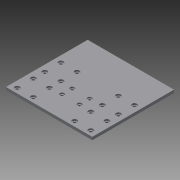
# Autodesk Inventor part: mic6_plate
Saved by Autodesk Inventor 2014 (Build 180170000, 170)
## iProperties
Created: 2014-08-09
Part Number: mic6_plate
Material: Generic
Document SubType Name: Modeling
Designer: Matthew
Density: 1 g/cm^3
Appearance: Default
Mass: 265.145 g
Surface Area: 932.163 cm^2
Volume: 265.145 cm^3
Author: Matthew
Autodesk Inventor part; units mm, degrees
ref_plane "YZ Plane" through (0, 0, 0) normal (1, 0, 0) x (0, 1, 0)
ref_plane "XZ Plane" through (0, 0, 0) normal (0, 1, 0) x (-1, 0, 0)
ref_plane "XY Plane" through (0, 0, 0) normal (0, 0, 1) x (1, 0, 0)
sketch "Sketch1" plane through (0, 0, 0) normal (0, 1, 0) x (-1, 0, 0)
  line L0 (93.9, 88.9) -> (-93.9, 88.9)
  line L1 (-93.9, 88.9) -> (-93.9, -88.9)
  line L2 (-93.9, -88.9) -> (93.9, -88.9)
  line L3 (93.9, -88.9) -> (93.9, 88.9)
  line L4 (93.9, 88.9) -> (-93.9, -88.9) construction
  line L5 (-93.9, 88.9) -> (93.9, -88.9) construction
  point P0 (0, 0)
  dimension "d0" = 187.8
  dimension "d1" = 177.8
  constraints: 12 end point, 2 midpoint, 2 parallel, 1 horizontal, 1 perpendicular
  measures "d0" distance of L2.end L1.end
  measures "d1" distance of L0.end L1.end
extrude "Extrusion1" add sketch "Sketch1" along normal blind 6.35
sketch "Sketch3" plane through (0, 6.35, 0) normal (0, 1, 0) x (1, 0, 0)
  line L0 (-93.9, 88.9) -> (-93.9, -88.9)
  line L1 (93.9, 88.9) -> (-93.9, 88.9)
  line L2 (-86.5034, 24.275) -> (-86.5034, -25.725) construction
  line L3 (-86.5034, -25.725) -> (-38.5034, -25.725) construction
  line L4 (-38.5034, -25.725) -> (-38.5034, 24.275) construction
  line L5 (-38.5034, 24.275) -> (-86.5034, 24.275) construction
  line L6 (38.5034, 24.275) -> (38.5034, -25.725) construction
  line L7 (38.5034, -25.725) -> (86.5034, -25.725) construction
  line L8 (86.5034, -25.725) -> (86.5034, 24.275) construction
  line L9 (86.5034, 24.275) -> (38.5034, 24.275) construction
  line L10 (-86.5034, -35.725) -> (-86.5034, -85.725) construction
  line L11 (-86.5034, -85.725) -> (-38.5034, -85.725) construction
  line L12 (-38.5034, -85.725) -> (-38.5034, -35.725) construction
  line L13 (-38.5034, -35.725) -> (-86.5034, -35.725) construction
  line L14 (38.5034, -35.725) -> (38.5034, -85.725) construction
  line L15 (38.5034, -85.725) -> (86.5034, -85.725) construction
  line L16 (86.5034, -85.725) -> (86.5034, -35.725) construction
  line L17 (86.5034, -35.725) -> (38.5034, -35.725) construction
  line L18 (-24, -13.225) -> (24, -13.225) construction
  line L19 (24, -13.225) -> (24, -48.225) construction
  line L20 (24, -48.225) -> (-24, -48.225) construction
  line L21 (-24, -48.225) -> (-24, -13.225) construction
  line L22 (93.9, -88.9) -> (93.9, 88.9) projected
  line L23 (-93.9, -88.9) -> (93.9, -88.9) projected
  point P0 (-133.35, 152.4)
  point P1 (-152.4, 133.35)
  point P2 (-152.4, -133.35)
  point P3 (133.35, 152.4)
  point P4 (0, -30.725)
  point P5 (-80.0034, 16.775)
  point P6 (-45.0034, 16.775)
  point P7 (-80.0034, -18.225)
  point P8 (-45.0034, -18.225)
  point P9 (45.0034, 16.775)
  point P10 (80.0034, 16.775)
  point P11 (45.0034, -18.225)
  point P12 (80.0034, -18.225)
  point P13 (-80.0034, -43.225)
  point P14 (-45.0034, -43.225)
  point P15 (-80.0034, -78.225)
  point P16 (-45.0034, -78.225)
  point P17 (45.0034, -43.225)
  point P18 (80.0034, -43.225)
  point P19 (45.0034, -78.225)
  point P20 (80.0034, -78.225)
  point P21 (0, -13.225)
  point P22 (62.5034, -30.725)
  point P23 (24, -30.725)
  point P24 (62.5034, 24.275)
  point P25 (-19, -19.725)
  point P26 (19, -19.725)
  point P27 (-19, -41.725)
  point P28 (19, -41.725)
  point P29 (-93.9, 88.9)
  dimension "d27" = 35
  dimension "d30" = 35
  dimension "d33" = 48
  dimension "d34" = 50
  dimension "d35" = 6.5
  dimension "d36" = 6.5
  dimension "d37" = 7.5
  dimension "d38" = 7.5
  dimension "d42" = 125.0068
  dimension "d45" = 60
  dimension "d50" = 48
  dimension "d51" = 35
  dimension "d52" = 5
  dimension "d53" = 6.5
  dimension "d56" = 38
  dimension "d59" = 22
  dimension "d78" = 14.5034
  dimension "d79" = 14.5034
  dimension "d80" = 10
  dimension "d81" = 5
  dimension "d82" = 173.0068
  dimension "d83" = 110
  dimension "d84" = 102.125
  dimension "d85" = 69.9
  dimension "d115" = 7.3966
  dimension "d116" = 7.3966
  dimension "d117" = 3.175
  constraints: 40 end point, 20 vertical alignment, 11 horizontal alignment, 10 parallel, 6 collinear, 3 midpoint, 2 horizontal, 2 perpendicular, 2 vertical, 9 other
  measures "d27" distance of point (-80.003, 16.775) point (-45.003, 16.775)
  measures "d30" distance of point (-80.003, 16.775) point (-80.003, -18.225)
  measures "d33" distance of L2.end L3.end
  measures "d34" distance of L3.end L4.end
  measures "d35" distance from line of L4 point (-45.003, 16.775)
  measures "d36" distance from line of L2 point (-80.003, 16.775)
  measures "d37" distance from line of L5 point (-45.003, 16.775)
  measures "d38" distance from line of L3 point (-45.003, -18.225)
  measures "d42" distance of L2.start L6.start
  measures "d45" distance of L2.start L10.start
  measures "d50" distance of L19.end L20.end
  measures "d51" distance of L18.end L19.end
  measures "d52" distance from line of L21 point (-19, -19.725)
  measures "d53" distance from line of L18 point (-19, -19.725)
  measures "d56" distance of point (-19, -19.725) point (19, -19.725)
  measures "d59" distance of point (-19, -19.725) point (-19, -41.725)
  measures "d78" distance between parallel lines of L21 L12
  measures "d79" distance between parallel lines of L14 L19
  measures "d80" distance between parallel lines of L7 L17
  measures "d81" distance from line of point (62.503, -30.725) L17
  measures "d82" distance between parallel lines of L16 L10
  measures "d83" distance between parallel lines of L15 L9
  measures "d115" distance between parallel lines of L22 L16
  measures "d117" distance between parallel lines of L23 L11
hole "Hole4" at (-80.0034, 6.35, 18.225) at (-80.0034, 6.35, -16.775) at (-80.0034, 6.35, 43.225) at (-80.0034, 6.35, 78.225) at (-45.0034, 6.35, 43.225) at (-45.0034, 6.35, 78.225) at (-45.0034, 6.35, 18.225) at (-45.0034, 6.35, -16.775) at (80.0034, 6.35, -16.775) at (80.0034, 6.35, 18.225) at (80.0034, 6.35, 43.225) at (80.0034, 6.35, 78.225) at (45.0034, 6.35, 78.225) at (45.0034, 6.35, 43.225) at (45.0034, 6.35, 18.225) at (45.0034, 6.35, -16.775) direction (0, -1, 0) diameter 6.6 end through all
hole "Hole5" at (-19, 6.35, 19.725) at (19, 6.35, 19.725) at (-19, 6.35, 41.725) at (19, 6.35, 41.725) direction (0, -1, 0) diameter 5.5 end through all
hole "Hole6" at (-80.0034, 6.35, -16.775) at (-45.0034, 6.35, -16.775) at (-45.0034, 6.35, 18.225) at (-80.0034, 6.35, 18.225) at (-80.0034, 6.35, 43.225) at (-45.0034, 6.35, 43.225) at (-45.0034, 6.35, 78.225) at (-80.0034, 6.35, 78.225) at (80.0034, 6.35, 78.225) at (80.0034, 6.35, 43.225) at (80.0034, 6.35, -16.775) at (80.0034, 6.35, 18.225) at (45.0034, 6.35, -16.775) at (45.0034, 6.35, 18.225) at (45.0034, 6.35, 78.225) at (45.0034, 6.35, 43.225) direction (0, -1, 0) diameter 10.6 depth 3.3
hole "Hole7" at (-19, 6.35, 19.725) at (19, 6.35, 19.725) at (19, 6.35, 41.725) at (-19, 6.35, 41.725) direction (0, -1, 0) diameter 9.6 depth 2.75
equation "\"d30\" = d27"
equation "\"d78\" = d79"
equation "\"d81\" = 0.5 * d80"
equation "\"d116\" = d115"
equation "\"d91\" = d59"
equation "\"d98\" = d59"
body "Solid1"
